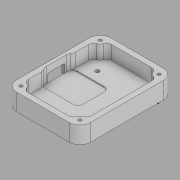
# Autodesk Inventor part: macropad-frame-v2
Saved by Autodesk Inventor 2019 (Build 230136000, 136)
## iProperties
Created: 2019-02-26
Part Number: macropad-frame-v2
Material: Generic
Document SubType Name: Modeling
Designer: onemo
Density: 1 g/cm^3
Appearance: Default
Author: onemo
Autodesk Inventor part; units mm, degrees
ref_plane "YZ Plane" through (0, 0, 0) normal (1, 0, 0) x (0, 1, 0)
ref_plane "XZ Plane" through (0, 0, 0) normal (0, 1, 0) x (-1, 0, 0)
ref_plane "XY Plane" through (0, 0, 0) normal (0, 0, 1) x (1, 0, 0)
sketch "Sketch1" plane through (0, 0, 0) normal (0, 1, 0) x (-1, 0, 0)
  line L0 (58.0321, 73.1889) -> (-11.1179, 73.1889)
  line L1 (-11.1179, 73.1889) -> (-11.1179, -15.0111)
  line L2 (-11.1179, -15.0111) -> (58.0321, -15.0111)
  line L3 (58.0321, -15.0111) -> (58.0321, 73.1889)
  point P0 (0, 0)
  dimension "d0" = 88.2
  dimension "d1" = 69.15
  constraints: 8 end point, 2 parallel, 1 horizontal, 1 perpendicular
  measures "d0" distance between parallel lines of L2 L0
  measures "d1" distance between parallel lines of L3 L1
extrude "Extrusion1" add sketch "Sketch1" along normal blind 3
sketch "Sketch2" plane through (0, 3, 0) normal (0, 1, 0) x (1, 0, 0)
  line L0 (-58.0321, -73.1889) -> (11.1179, -73.1889) projected
  line L1 (11.1179, -73.1889) -> (11.1179, 15.0111) projected
  line L2 (-58.0321, -73.1889) -> (11.1179, -73.1889)
  line L3 (11.1179, -73.1889) -> (11.1179, 15.0111)
  line L4 (11.1179, 15.0111) -> (-58.0321, 15.0111)
  line L5 (-58.0321, 15.0111) -> (-58.0321, -73.1889)
  line L6 (-53.0321, -68.1889) -> (6.1179, -68.1889)
  line L7 (6.1179, -68.1889) -> (6.1179, 10.0111)
  line L8 (6.1179, 10.0111) -> (-53.0321, 10.0111)
  line L9 (-53.0321, 10.0111) -> (-53.0321, -68.1889)
  line L10 (-58.0321, 15.0111) -> (-58.0321, -73.1889) projected
  line L11 (-58.0321, -73.1889) -> (-47.0321, -73.1889)
  line L12 (-47.0321, -73.1889) -> (-47.0321, -62.1889)
  line L13 (-47.0321, -62.1889) -> (-58.0321, -62.1889)
  line L14 (-58.0321, -62.1889) -> (-58.0321, -73.1889)
  line L15 (-58.0321, 15.0111) -> (-47.0321, 15.0111)
  line L16 (-47.0321, 15.0111) -> (-47.0321, 4.0111)
  line L17 (-47.0321, 4.0111) -> (-58.0321, 4.0111)
  line L18 (-58.0321, 4.0111) -> (-58.0321, 15.0111)
  line L19 (11.1179, 15.0111) -> (0.1179, 15.0111)
  line L20 (0.1179, 15.0111) -> (0.1179, 4.0111)
  line L21 (0.1179, 4.0111) -> (11.1179, 4.0111)
  line L22 (11.1179, 4.0111) -> (11.1179, 15.0111)
  line L23 (11.1179, -73.1889) -> (0.1179, -73.1889)
  line L24 (0.1179, -73.1889) -> (0.1179, -62.1889)
  line L25 (0.1179, -62.1889) -> (11.1179, -62.1889)
  line L26 (11.1179, -62.1889) -> (11.1179, -73.1889)
  arc A0 (1.3427, -62.1889) -> (6.1179, -57.4137) centre (1.3427, -57.4137) ccw
  arc A1 (-4.6573, -68.1889) -> (0.1179, -63.4137) centre (-4.6573, -63.4137) ccw
  arc A2 (-47.0321, -63.4137) -> (-42.2569, -68.1889) centre (-42.2569, -63.4137) ccw
  arc A3 (-53.0321, -57.4137) -> (-48.2569, -62.1889) centre (-48.2569, -57.4137) ccw
  arc A4 (-48.2569, 4.0111) -> (-53.0321, -0.7641) centre (-48.2569, -0.7641) ccw
  arc A5 (-42.2569, 10.0111) -> (-47.0321, 5.2359) centre (-42.2569, 5.2359) ccw
  arc A6 (0.1179, 5.2359) -> (-4.6573, 10.0111) centre (-4.6573, 5.2359) ccw
  arc A7 (6.1179, -0.7641) -> (1.3427, 4.0111) centre (1.3427, -0.7641) ccw
  point P0 (0, 0)
  dimension "d4" = 5
  dimension "d5" = 5
  dimension "d6" = 5
  dimension "d7" = 5
  dimension "d8" = 6
  dimension "d9" = 6
  dimension "d10" = 6
  dimension "d11" = 6
  dimension "d12" = 6
  dimension "d13" = 6
  dimension "d14" = 6
  dimension "d15" = 6
  dimension "d16" = 4.7752
  dimension "d17" = 4.7752
  dimension "d18" = 4.7752
  dimension "d19" = 4.7752
  dimension "d20" = 4.7752
  dimension "d21" = 4.7752
  dimension "d22" = 4.7752
  dimension "d23" = 4.7752
  dimension "d24" = 4.7752
  dimension "d25" = 4.7752
  dimension "d26" = 4.7752
  dimension "d27" = 4.7752
  dimension "d28" = 4.7752
  dimension "d29" = 4.7752
  dimension "d30" = 4.7752
  dimension "d31" = 4.7752
  dimension "d32" = 4.7752
  dimension "d33" = 4.7752
  dimension "d34" = 4.7752
  dimension "d35" = 4.7752
  dimension "d36" = 4.7752
  dimension "d37" = 4.7752
  dimension "d38" = 4.7752
  dimension "d39" = 4.7752
  constraints: 48 end point, 17 point on line, 16 point on circle, 12 parallel, 8 centre point, 6 horizontal, 6 perpendicular, 1 tangent
  measures "d4" distance between parallel lines of L6 L0
  measures "d5" distance between parallel lines of L4 L8
  measures "d6" distance between parallel lines of L7 L1
  measures "d7" distance between parallel lines of L5 L9
  measures "d8" distance between parallel lines of L13 L6
  measures "d9" distance between parallel lines of L12 L9
  measures "d10" distance between parallel lines of L7 L24
  measures "d11" distance between parallel lines of L6 L25
  measures "d12" distance between parallel lines of L8 L21
  measures "d13" distance between parallel lines of L20 L7
  measures "d14" distance between parallel lines of L8 L17
  measures "d15" distance from line of L9 L16.end
  measures "d16" radius of A0
  measures "d17" radius of A1
  measures "d18" radius of A2
  measures "d19" radius of A3
  measures "d20" distance from line of L25 A0.end
  measures "d21" distance from line of L7 A0.start
  measures "d22" distance from line of L6 A1.end
  measures "d23" distance from line of L24 A1.start
  measures "d24" distance from line of L13 A3.start
  measures "d25" distance from line of L9 A3.end
  measures "d26" distance from line of L12 A2.end
  measures "d27" distance from line of L6 A2.start
  measures "d28" distance from line of L9 A4.start
  measures "d29" distance from line of L17 A4.end
  measures "d30" radius of A4
  measures "d31" distance from line of L8 A5.end
  measures "d32" distance from line of L16 A5.start
  measures "d33" radius of A5
  measures "d34" distance from line of L8 A6.start
  measures "d35" distance from line of L20 A6.end
  measures "d36" radius of A6
  measures "d37" distance from line of L7 A7.end
  measures "d38" distance from line of L21 A7.start
  measures "d39" radius of A7
extrude "Extrusion3" add sketch "Sketch2" along normal blind 13 contours L5 L13 L9 L6 L12 L0 | L12 L6 L24 L0 | L5 L17 L9 L13 | L24 L6 L7 L25 L1 L0 | L12 A2 L6 | L6 L9 L13 L12 | L5 L4 L16 L8 L9 L17 | L9 A3 L13 | L24 L25 L7 L6 | L6 A1 L24 | L17 A4 L9 | L9 L8 L16 L17 | L25 L7 L21 L1 | L4 L20 L8 L16 | L21 L7 L8 L20 L4 L1 | L25 A0 L7 | L8 A5 L16 | L21 L20 L8 L7 | L7 A7 L21 | L20 A6 L8
fillet "Fillet1" radius 4.7752 4 edges at (0.1179, 9.5, 62.1889) (-47.0321, 9.5, 62.1889) (-47.0321, 9.5, -4.0111) (0.1179, 9.5, -4.0111)
fillet "Fillet2" radius 10 4 edges at (11.1179, 8, 73.1889) (-58.0321, 8, 73.1889) (11.1179, 8, -15.0111) (-58.0321, 8, -15.0111)
sketch "Sketch4" plane through (11.1179, 0, 63.1889) normal (1, 0, 0) x (0, 0, -1)
  point P0 (63.1889, 0)
sketch "Sketch5" plane through (-58.0321, 0, -5.0111) normal (-1, 0, 0) x (0, 0, 1)
  line L0 (68.2, 0) -> (0, 0) projected
  line L1 (42.2, 0) -> (26, 0)
  line L2 (26, 0) -> (26, 10)
  line L3 (26, 10) -> (42.2, 10)
  line L4 (42.2, 10) -> (42.2, 0)
  line L5 (78.2, 0) -> (78.2, 16) projected
  line L6 (-10, 16) -> (-10, 0) projected
  arc A0 (42.2, 8.73) -> (40.93, 10) centre (40.5854, 8.3854) ccw
  arc A1 (27.27, 10) -> (26, 8.73) centre (27.6146, 8.3854) ccw
  point P0 (5.0111, 0)
  dimension "d48" = 10
  dimension "d49" = 16.2
  dimension "d50" = 1.27
  dimension "d51" = 1.27
  dimension "d52" = 1.27
  dimension "d53" = 1.27
  dimension "d54" = 1.651
  dimension "d55" = 1.651
  dimension "d58" = 88.2
  dimension "d59" = 36
  dimension "d60" = 36
  constraints: 8 end point, 5 point on line, 4 point on circle, 2 centre point, 2 parallel, 1 horizontal, 1 perpendicular
  measures "d48" distance between parallel lines of L0 L3
  measures "d49" distance between parallel lines of L2 L4
  measures "d50" distance from line of L4 A0.end
  measures "d51" distance from line of L3 A0.start
  measures "d52" distance from line of L2 A1.start
  measures "d53" distance from line of L3 A1.end
  measures "d54" radius of A0
  measures "d55" radius of A1
  measures "d58" distance between parallel lines of L6 L5
  measures "d59" distance between parallel lines of L5 L4
  measures "d60" distance between parallel lines of L6 L2
extrude "Extrusion4" cut sketch "Sketch5" against normal blind 3 contours L0 L2 A1 L3 A0 L4
sketch "Sketch7" plane through (0, 16, 0) normal (0, 1, 0) x (1, 0, 0)
  line L0 (-53.0321, -0.7641) -> (-53.0321, -57.4137) projected
  line L1 (-53.0321, -43.5889) -> (-55.0321, -43.5889)
  line L2 (-55.0321, -43.5889) -> (-55.0321, -14.5889)
  line L3 (-55.0321, -14.5889) -> (-53.0321, -14.5889)
  line L4 (-53.0321, -14.5889) -> (-53.0321, -43.5889)
  line L5 (-48.0321, -73.1889) -> (1.1179, -73.1889) projected
  line L6 (1.1179, 15.0111) -> (-48.0321, 15.0111) projected
  line L7 (-55.0321, -43.5889) -> (-20.0321, -43.5889)
  line L8 (-20.0321, -43.5889) -> (-20.0321, -14.5889)
  line L9 (-20.0321, -14.5889) -> (-55.0321, -14.5889)
  line L10 (-55.0321, -14.5889) -> (-55.0321, -43.5889)
  arc A0 (-55.0321, -38.5089) -> (-49.9521, -43.5889) centre (-50.2673, -38.8241) ccw
  arc A1 (-49.9521, -14.5889) -> (-55.0321, -19.6689) centre (-50.2673, -19.3536) ccw
  arc A2 (-25.1121, -43.5889) -> (-20.0321, -38.5089) centre (-24.7969, -38.8241) ccw
  arc A3 (-20.0321, -19.6689) -> (-25.1121, -14.5889) centre (-24.7969, -19.3536) ccw
  point P0 (0, 0)
  dimension "d61" = 29.6
  dimension "d62" = 88.2
  dimension "d63" = 29
  dimension "d64" = 2
  dimension "d65" = 35
  dimension "d66" = 5.08
  dimension "d67" = 5.08
  dimension "d68" = 5.08
  dimension "d69" = 5.08
  dimension "d70" = 5.08
  dimension "d71" = 5.08
  dimension "d72" = 5.08
  dimension "d73" = 5.08
  dimension "d75" = 4.7752
  dimension "d76" = 4.7752
  dimension "d77" = 4.7752
  dimension "d78" = 29
  dimension "d82" = 4.7752
  dimension "d107" = 18.84
  constraints: 16 end point, 9 point on line, 8 point on circle, 4 centre point, 4 parallel, 2 horizontal, 2 perpendicular
  measures "d61" distance between parallel lines of L5 L1
  measures "d62" distance between parallel lines of L6 L5
  measures "d63" distance between parallel lines of L3 L1
  measures "d64" distance between parallel lines of L2 L0
  measures "d65" distance between parallel lines of L2 L8
  measures "d66" distance of L1.end A0.end
  measures "d67" distance from line of L7 A0.start
  measures "d68" distance from line of L3 A1.end
  measures "d69" distance from line of L2 A1.start
  measures "d70" distance from line of L8 A3.end
  measures "d71" distance from line of L9 A3.start
  measures "d72" distance from line of L8 A2.start
  measures "d73" distance from line of L7 A2.end
  measures "d75" radius of A3
  measures "d76" radius of A0
  measures "d77" radius of A1
  measures "d78" distance between parallel lines of L9 L7
  measures "d82" radius of A2
  measures "d107" distance of A1.end A0.start
extrude "Extrusion5" cut sketch "Sketch7" against normal blind 14 contours A1 L9 A3 L8 A2 L7 A0 L0 | L0 A0 L2 A1 | A1 L9 | L2 A1 | A0 L2 | L7 A0 | A3 L9 | L7 A2 | A3 L8 | L8 A2
fillet "Fillet3" radius 4.7752 2 edges at (-53.0321, 9.5, 42.7175) (-53.0321, 9.5, 15.4602)
sketch "Sketch8" plane through (0, 16, 0) normal (0, 1, 0) x (1, 0, 0)
  line L0 (-48.0321, -73.1889) -> (1.1179, -73.1889) projected
  line L1 (-58.0321, 5.0111) -> (-58.0321, -63.1889) projected
  line L2 (11.1179, -63.1889) -> (11.1179, 5.0111) projected
  line L3 (1.1179, 15.0111) -> (-48.0321, 15.0111) projected
  point P0 (0, 0)
  point P1 (-51.0321, 8.0111)
  point P2 (4.1179, 8.0111)
  point P3 (4.1179, -66.1889)
  point P4 (-51.0321, -66.1889)
  dimension "d83" = 7
  dimension "d84" = 7
  dimension "d85" = 7
  dimension "d86" = 7
  dimension "d87" = 7
  dimension "d88" = 7
  dimension "d89" = 7
  dimension "d90" = 7
  measures "d83" distance from line of L0 point (-51.032, -66.189)
  measures "d84" distance from line of L1 point (-51.032, -66.189)
  measures "d85" distance from line of L0 point (4.118, -66.189)
  measures "d86" distance from line of L2 point (4.118, -66.189)
  measures "d87" distance from line of L2 point (4.118, 8.011)
  measures "d88" distance from line of L3 point (4.118, 8.011)
  measures "d89" distance from line of L3 point (-51.032, 8.011)
  measures "d90" distance from line of L1 point (-51.032, 8.011)
hole "Hole1" at (-51.0321, 16, -8.0111) at (4.1179, 16, -8.0111) at (4.1179, 16, 66.1889) at (-51.0321, 16, 66.1889) direction (0, -1, 0) diameter 3 depth 10
sketch "Sketch9" plane through (0, 3, 0) normal (0, 1, 0) x (1, 0, 0)
  line L0 (1.1179, 15.0111) -> (-48.0321, 15.0111) projected
  line L1 (-58.0321, 5.0111) -> (-58.0321, -63.1889) projected
  point P0 (0, 0)
  point P1 (-40.2521, -5.3089)
  dimension "d98" = 20.32
  dimension "d99" = 17.78
  measures "d98" distance from line of L0 point (-40.252, -5.309)
  measures "d99" distance from line of L1 point (-40.252, -5.309)
hole "Hole2" at (-40.2521, 3, 5.3089) direction (0, -1, 0) diameter 3.75 depth 10
equation "\"d5\" = d4"
equation "\"d6\" = d4"
equation "\"d7\" = d4"
equation "\"d9\" = d8"
equation "\"d10\" = d8"
equation "\"d11\" = d8"
equation "\"d12\" = d8"
equation "\"d14\" = d8"
equation "\"d15\" = d9"
equation "\"d17\" = d16"
equation "\"d18\" = d16"
equation "\"d19\" = d18"
equation "\"d25\" = d24"
equation "\"d26\" = d25"
equation "\"d27\" = d25"
equation "\"d28\" = d21"
equation "\"d29\" = d28"
equation "\"d30\" = d16"
equation "\"d31\" = d28"
equation "\"d32\" = d31"
equation "\"d33\" = d30"
equation "\"d34\" = d31"
equation "\"d35\" = d34"
equation "\"d36\" = d33"
equation "\"d37\" = d34"
equation "\"d38\" = d37"
equation "\"d39\" = d36"
equation "\"d51\" = d50"
equation "\"d52\" = d50"
equation "\"d53\" = d50"
equation "\"d54\" = d55"
equation "\"d59\" = -0.5 * d49 + 0.5 * d58"
equation "\"d61\" = -0.5 * d63 + 0.5 * d62"
equation "\"d67\" = d66"
equation "\"d68\" = d67"
equation "\"d69\" = d68"
equation "\"d70\" = d67"
equation "\"d71\" = d70"
equation "\"d72\" = d73"
equation "\"d73\" = d71"
equation "\"d76\" = d74"
equation "\"d77\" = d74"
equation "\"d78\" = d63"
equation "\"d82\" = d75"
equation "\"d84\" = d83"
equation "\"d85\" = d83"
equation "\"d86\" = d83"
equation "\"d87\" = d83"
equation "\"d88\" = d87"
equation "\"d89\" = d88"
equation "\"d90\" = d88"
equation "\"d74\" = 4.7752"
body "Solid1"
